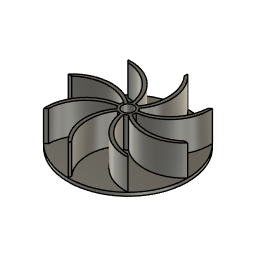
Rotor v3 (Autodesk Fusion 360 design; units mm, degrees)
Autodesk Fusion 360 part; units mm, degrees
sketch "Skizze1" plane through (0, 0, 0) normal (0, 0, 1) x (1, 0, 0)
  line L0 (-9.3696, -9.3689) -> (-13.6122, -5.1262) construction
  line L1 (-0.0006, -13.2498) -> (-4.5006, -13.2498) construction
  line L2 (-0.0004, 0) -> (18.7379, -18.7383)
  line L3 (-0.0004, 0) -> (18.7379, -18.7383) construction
  line L4 (-18.7387, -18.738) -> (-17.6781, -17.6774) construction
  arc A0 (-0.0006, -24.9998) -> (-0.0006, -1.4998) centre (13.0897, -13.2498) cw
  line L5 (13.2496, 0) -> (13.2496, -6) construction
  line L6 (-0.0006, -26.4998) -> (-0.0006, -24.9998) construction
  line L7 (-9.3696, 9.3692) -> (-5.1269, 13.6118) construction
  line L8 (-9.3696, 9.3692) -> (-5.1269, 13.6118) construction
  line L9 (-9.3696, 9.3692) -> (-6.1876, 12.5511) construction
  line L10 (-9.3696, 9.3692) -> (-6.1876, 12.5511) construction
  line L11 (-9.3696, 9.3692) -> (-6.1876, 12.5511) construction
  line L12 (-0.0004, 0) -> (18.7379, -18.7383) construction
  line L13 (-9.3696, 9.3692) -> (-5.1269, 13.6118) construction
  line L14 (9.3687, -9.3692) -> (5.1261, -13.6118) construction
  line L15 (9.3687, -9.3692) -> (6.1868, -12.5511) construction
  line L16 (9.3687, -9.3692) -> (6.1868, -12.5511) construction
  line L17 (9.3687, -9.3692) -> (5.1261, -13.6118) construction
  line L18 (9.3687, -9.3692) -> (6.1868, -12.5511) construction
  line L19 (-0.0006, -13.2498) -> (-6.0006, -13.2498) construction
  arc A1 (-17.6781, -17.6774) -> (-1.0611, -1.0604) centre (-0.1134, -18.6251) cw
  line L20 (9.3687, -9.3692) -> (6.1868, -12.5511) construction
  line L21 (9.3687, -9.3692) -> (5.1261, -13.6118) construction
  line L22 (9.3687, -9.3692) -> (5.1261, -13.6118) construction
  line L23 (9.3687, -9.3692) -> (5.1261, -13.6118) construction
  line L24 (9.3687, -9.3692) -> (6.1868, -12.5511) construction
  line L25 (-9.3696, -9.3689) -> (-12.5516, -6.1869) construction
  line L26 (-18.7387, 18.7383) -> (-17.6781, 17.6777) construction
  line L27 (-18.7387, 18.7383) -> (-17.6781, 17.6777) construction
  arc A2 (26.4996, 0) -> (-0.0004, 0) centre (13.2496, 11.6302) cw
  arc A3 (-25.0004, 0) -> (-1.5004, 0) centre (-13.2504, -13.0903) cw
  line L28 (-13.2504, 0) -> (-13.2504, 4.5) construction
  line L29 (-13.2504, 0) -> (-13.2504, 6) construction
  line L30 (-13.2504, 0) -> (-13.2504, 6) construction
  arc A4 (-25.0004, 0) -> (-1.5004, 0) centre (-13.2504, -13.0903) cw
  line L31 (-26.5004, 0) -> (-25.0004, 0) construction
  line L32 (-26.5004, 0) -> (-25.0004, 0) construction
  arc A5 (-17.6781, 17.6777) -> (-1.0611, 1.0607) centre (-18.6258, 0.1129) cw
  line L33 (-26.5004, 0) -> (-25.0004, 0) construction
  line L34 (-18.7387, 18.7383) -> (-17.6781, 17.6777) construction
  line L35 (-18.7387, 18.7383) -> (-17.6781, 17.6777) construction
  line L36 (-26.5004, 0) -> (-25.0004, 0) construction
  line L37 (-9.3696, 9.3692) -> (-5.1269, 13.6118) construction
  line L38 (-9.3696, 9.3692) -> (-6.1876, 12.5511) construction
  line L39 (-26.5004, 0) -> (-25.0004, 0) construction
  line L40 (-9.3696, 9.3692) -> (-5.1269, 13.6118) construction
  line L41 (-9.3696, 9.3692) -> (-6.1876, 12.5511) construction
  line L42 (-18.7387, 18.7383) -> (-17.6781, 17.6777) construction
  line L43 (-0.0004, 0) -> (-18.7387, 18.7383)
  line L44 (-0.0004, 0) -> (-1.0611, 1.0607) construction
  line L45 (-0.0004, 0) -> (-26.5004, 0)
  line L46 (-0.0004, 0) -> (-18.7387, 18.7383)
  line L47 (-0.0004, 0) -> (-1.0611, 1.0607) construction
  line L48 (-0.0004, 0) -> (-26.5004, 0)
  line L49 (-0.0004, 0) -> (13.2496, 0) construction
  line L50 (-0.0004, 0) -> (-26.5004, 0) construction
  line L51 (-0.0004, 0) -> (-9.3696, 9.3692) construction
  line L52 (-0.0004, 0) -> (-1.5004, 0) construction
  line L53 (-0.0004, 0) -> (-13.2504, 0) construction
  line L54 (-0.0004, 0) -> (26.4996, 0) construction
  arc A6 (-26.5004, 0) -> (-0.0004, 0) centre (-13.2504, -11.6302) cw
  line L55 (-0.0004, 0) -> (-26.5004, 0) construction
  line L56 (-0.0004, 0) -> (-9.3696, 9.3692) construction
  line L57 (-0.0004, 0) -> (-9.3696, 9.3692) construction
  line L58 (13.2496, 0) -> (13.2496, -4.5) construction
  line L59 (-0.0004, 0) -> (1.4996, 0) construction
  circle A7 centre (-0.0004, 0) radius 26.5
  line L60 (-0.0004, 0) -> (9.3687, -9.3692) construction
  line L61 (-0.0004, 0) -> (18.7379, -18.7383) construction
  line L62 (-0.0004, 0) -> (-9.3696, 9.3692) construction
  line L63 (-0.0002, -0.0002) -> (-0.0002, 26.4998)
  line L64 (-0.0004, 0) -> (-1.0611, 1.0607) construction
  circle A8 centre (-0.0004, 0) radius 2.55
  arc A9 (-18.7387, 18.7383) -> (-0.0004, 0) centre (-17.5934, 1.1454) cw
  line L65 (-0.0004, 0) -> (1.4996, 0) construction
  line L66 (-0.0004, 0) -> (26.4996, 0)
  line L67 (-0.0004, 0) -> (13.2496, 0) construction
  line L68 (-0.0004, 0) -> (26.4996, 0)
  line L69 (-0.0004, 0) -> (-1.0611, 1.0607) construction
  arc A10 (-0.0002, 24.9998) -> (-0.0002, 1.4998) centre (-13.0905, 13.2498) cw
  line L70 (-0.0004, 0.0003) -> (-9.3696, -9.3689) construction
  line L71 (-0.0004, 0) -> (-18.7387, 18.7383) construction
  line L72 (-0.0004, -0.0003) -> (9.3687, 9.3689) construction
  arc A11 (-0.0002, 26.4998) -> (-0.0002, -0.0002) centre (-11.6304, 13.2498) cw
  line L73 (-0.0004, 0) -> (-26.5004, 0)
  line L74 (-0.0004, 0) -> (-26.5004, 0)
  line L75 (-0.0004, 0) -> (-26.5004, 0) construction
  arc A12 (-26.5004, 0) -> (-0.0004, 0) centre (-13.2504, -11.6302) cw
  arc A13 (-18.7387, 18.7383) -> (-0.0004, 0) centre (-17.5934, 1.1454) cw
  line L76 (-0.0004, 0) -> (26.4996, 0) construction
  line L77 (-0.0004, 0) -> (26.4996, 0) construction
  line L78 (-0.0004, 0) -> (-26.5004, 0) construction
  line L79 (-0.0004, 0) -> (-26.5004, 0)
  arc A14 (18.7379, 18.738) -> (-0.0004, -0.0003) centre (1.1449, 17.5927) cw
  line L80 (-0.0004, 0) -> (1.4996, 0) construction
  arc A15 (-26.5004, 0) -> (-0.0004, 0) centre (-13.2504, -11.6302) cw
  line L81 (-0.0004, 0) -> (-18.7387, 18.7383) construction
  line L82 (-0.0004, 0) -> (26.4996, 0)
  line L83 (-0.0004, 0) -> (-26.5004, 0) construction
  line L84 (-0.0004, 0) -> (26.4996, 0)
  arc A16 (-18.7387, 18.7383) -> (-0.0004, 0) centre (-17.5934, 1.1454) cw
  arc A17 (-18.7387, 18.7383) -> (-0.0004, 0) centre (-17.5934, 1.1454) cw
  line L85 (-0.0004, 0) -> (-1.5004, 0) construction
  line L86 (-0.0004, 0) -> (-13.2504, 0) construction
  line L87 (-0.0004, 0) -> (-1.5004, 0) construction
  line L88 (-0.0004, 0) -> (26.4996, 0) construction
  line L89 (-0.0004, 0) -> (-13.2504, 0) construction
  line L90 (-0.0004, 0) -> (1.4996, 0) construction
  arc A18 (-18.7387, 18.7383) -> (-0.0004, 0) centre (-17.5934, 1.1454) cw
  line L91 (-0.0004, 0) -> (13.2496, 0) construction
  line L92 (-0.0004, 0) -> (-18.7387, 18.7383)
  line L93 (-0.0004, 0) -> (-18.7387, 18.7383) construction
  line L94 (-0.0004, 0) -> (26.4996, 0) construction
  line L95 (-0.0004, 0) -> (-1.5004, 0) construction
  line L96 (-0.0004, 0) -> (-1.5004, 0) construction
  line L97 (-0.0004, 0) -> (-18.7387, 18.7383) construction
  arc A19 (-26.5004, 0) -> (-0.0004, 0) centre (-13.2504, -11.6302) cw
  line L98 (-0.0004, 0) -> (1.4996, 0) construction
  line L99 (-0.0004, 0) -> (-13.2504, 0) construction
  arc A20 (-26.5004, 0) -> (-0.0004, 0) centre (-13.2504, -11.6302) cw
  line L100 (-0.0004, 0) -> (-18.7387, 18.7383)
  line L101 (-0.0004, 0) -> (-18.7387, 18.7383) construction
  line L102 (-0.0004, 0) -> (-9.3696, 9.3692) construction
  line L103 (-0.0004, 0) -> (-13.2504, 0) construction
  line L104 (-0.0004, 0) -> (-18.7387, 18.7383)
  line L105 (-0.0004, 0) -> (-1.0611, 1.0607) construction
  line L106 (-0.0004, 0) -> (13.2496, 0) construction
  line L107 (-0.0004, 0) -> (13.2496, 0) construction
  line L108 (-0.0004, 0) -> (26.4996, 0)
  arc A21 (17.6773, -17.6777) -> (1.0602, -1.0607) centre (18.625, -0.1129) cw
  line L109 (18.7379, -18.7383) -> (17.6773, -17.6777) construction
  arc A22 (17.6773, -17.6777) -> (1.0602, -1.0607) centre (18.625, -0.1129) cw
  arc A23 (17.6773, -17.6777) -> (1.0602, -1.0607) centre (18.625, -0.1129) cw
  arc A24 (17.6773, -17.6777) -> (1.0602, -1.0607) centre (18.625, -0.1129) cw
  arc A25 (17.6773, -17.6777) -> (1.0602, -1.0607) centre (18.625, -0.1129) cw
  line L110 (18.7379, -18.7383) -> (17.6773, -17.6777) construction
  line L111 (18.7379, -18.7383) -> (17.6773, -17.6777) construction
  line L112 (18.7379, -18.7383) -> (17.6773, -17.6777) construction
  line L113 (18.7379, -18.7383) -> (17.6773, -17.6777) construction
  arc A26 (-25.0004, 0) -> (-1.5004, 0) centre (-13.2504, -13.0903) cw
  arc A27 (-17.6781, 17.6777) -> (-1.0611, 1.0607) centre (-18.6258, 0.1129) cw
  line L114 (13.2496, 0) -> (13.2496, -4.5) construction
  line L115 (13.2496, 0) -> (13.2496, -6) construction
  arc A28 (26.4996, 0) -> (-0.0004, 0) centre (13.2496, 11.6302) cw
  line L116 (-13.2504, 0) -> (-13.2504, 4.5) construction
  line L117 (-0.0004, 0) -> (18.7379, -18.7383) construction
  arc A29 (-17.6781, 17.6777) -> (-1.0611, 1.0607) centre (-18.6258, 0.1129) cw
  arc A30 (-18.7387, -18.738) -> (-0.0004, 0.0003) centre (-1.1458, -17.5927) cw
  line L118 (-13.2504, 0) -> (-13.2504, 4.5) construction
  arc A31 (-25.0004, 0) -> (-1.5004, 0) centre (-13.2504, -13.0903) cw
  line L119 (-13.2504, 0) -> (-13.2504, 6) construction
  line L120 (-0.0004, 0) -> (9.3687, -9.3692) construction
  arc A32 (-17.6781, 17.6777) -> (-1.0611, 1.0607) centre (-18.6258, 0.1129) cw
  line L121 (-13.2504, 0) -> (-13.2504, 6) construction
  arc A33 (-17.6781, 17.6777) -> (-1.0611, 1.0607) centre (-18.6258, 0.1129) cw
  arc A34 (26.4996, 0) -> (-0.0004, 0) centre (13.2496, 11.6302) cw
  arc A35 (18.7379, -18.7383) -> (-0.0004, 0) centre (17.5925, -1.1454) cw
  circle A36 centre (-0.0004, 0) radius 3.5
  line L122 (-13.2504, 0) -> (-13.2504, 6) construction
  line L123 (-0.0004, 0.0003) -> (-18.7387, -18.738)
  line L124 (13.2496, 0) -> (13.2496, -4.5) construction
  line L125 (-0.0004, 0) -> (18.7379, -18.7383) construction
  line L126 (-13.2504, 0) -> (-13.2504, 4.5) construction
  arc A37 (-25.0004, 0) -> (-1.5004, 0) centre (-13.2504, -13.0903) cw
  line L127 (-13.2504, 0) -> (-13.2504, 4.5) construction
  line L128 (-0.0004, 0) -> (18.7379, -18.7383)
  line L129 (-0.0004, 0) -> (18.7379, -18.7383)
  line L130 (-0.0004, 0) -> (1.0602, -1.0607) construction
  line L131 (-0.0004, -0.0003) -> (1.0602, 1.0604) construction
  arc A38 (24.9996, 0) -> (1.4996, 0) centre (13.2496, 13.0903) cw
  line L132 (26.4996, 0) -> (24.9996, 0) construction
  line L133 (13.2496, 0) -> (13.2496, -4.5) construction
  arc A39 (-0.0006, -26.4998) -> (-0.0006, 0.0002) centre (11.6296, -13.2498) cw
  line L134 (-0.0002, 26.4998) -> (-0.0002, 24.9998) construction
  arc A40 (18.7379, -18.7383) -> (-0.0004, 0) centre (17.5925, -1.1454) cw
  line L135 (13.2496, 0) -> (13.2496, -4.5) construction
  line L136 (26.4996, 0) -> (24.9996, 0) construction
  line L137 (-0.0006, 0.0002) -> (-0.0006, -1.4998) construction
  arc A41 (26.4996, 0) -> (-0.0004, 0) centre (13.2496, 11.6302) cw
  line L138 (-0.0006, 0.0002) -> (-0.0006, -26.4998) construction
  line L139 (13.2496, 0) -> (13.2496, -6) construction
  line L140 (26.4996, 0) -> (24.9996, 0) construction
  line L141 (-0.0004, 0) -> (1.0602, -1.0607) construction
  line L142 (-0.0002, -0.0002) -> (-0.0002, 1.4998) construction
  line L143 (-0.0004, 0) -> (18.7379, -18.7383)
  line L144 (-0.0004, 0) -> (9.3687, -9.3692) construction
  arc A42 (24.9996, 0) -> (1.4996, 0) centre (13.2496, 13.0903) cw
  line L145 (-0.0004, 0) -> (1.0602, -1.0607) construction
  line L146 (-0.0006, 0.0002) -> (-0.0006, -26.4998)
  line L147 (26.4996, 0) -> (24.9996, 0) construction
  line L148 (-0.0004, 0) -> (1.0602, -1.0607) construction
  line L149 (26.4996, 0) -> (24.9996, 0) construction
  arc A43 (18.7379, -18.7383) -> (-0.0004, 0) centre (17.5925, -1.1454) cw
  line L150 (-0.0002, -0.0002) -> (-0.0002, 13.2498) construction
  arc A44 (17.6773, 17.6774) -> (1.0602, 1.0604) centre (0.1125, 18.6251) cw
  arc A45 (18.7379, -18.7383) -> (-0.0004, 0) centre (17.5925, -1.1454) cw
  arc A46 (26.4996, 0) -> (-0.0004, 0) centre (13.2496, 11.6302) cw
  line L151 (18.7379, 18.738) -> (17.6773, 17.6774) construction
  line L152 (-0.0004, 0) -> (1.0602, -1.0607) construction
  line L153 (-0.0004, 0.0003) -> (-1.0611, -1.0604) construction
  line L154 (-0.0004, 0.0003) -> (-18.7387, -18.738) construction
  line L155 (-0.0004, 0) -> (9.3687, -9.3692) construction
  line L156 (-0.0004, 0) -> (9.3687, -9.3692) construction
  line L157 (-0.0002, 13.2498) -> (4.4998, 13.2498) construction
  line L158 (-0.0006, 0.0002) -> (-0.0006, -13.2498) construction
  line L159 (-0.0002, -0.0002) -> (-0.0002, 26.4998) construction
  arc A47 (24.9996, 0) -> (1.4996, 0) centre (13.2496, 13.0903) cw
  line L160 (9.3687, 9.3689) -> (13.6114, 5.1262) construction
  arc A48 (18.7379, -18.7383) -> (-0.0004, 0) centre (17.5925, -1.1454) cw
  arc A49 (24.9996, 0) -> (1.4996, 0) centre (13.2496, 13.0903) cw
  line L161 (9.3687, 9.3689) -> (12.5507, 6.1869) construction
  line L162 (13.2496, 0) -> (13.2496, -6) construction
  line L163 (-0.0002, 13.2498) -> (5.9998, 13.2498) construction
  line L164 (-0.0004, -0.0003) -> (18.7379, 18.738) construction
  line L165 (-0.0004, -0.0003) -> (18.7379, 18.738)
  line L166 (-0.0004, 0) -> (18.7379, -18.7383)
  line L167 (13.2496, 0) -> (13.2496, -6) construction
  arc A50 (24.9996, 0) -> (1.4996, 0) centre (13.2496, 13.0903) cw
  point P0 (-0.0006, 0.0002)
  point P1 (-0.0004, 0)
  point P2 (-0.0004, 0)
  point P3 (-0.0006, 0.0002)
  point P4 (-0.0006, 0.0002)
  point P5 (-0.0004, 0)
  point P6 (-0.0004, 0)
  point P7 (-0.0004, 0)
  point P8 (-0.0004, 0)
  point P9 (-0.0004, 0)
  point P10 (-0.0004, 0)
  point P11 (-0.0004, 0)
  point P12 (-0.0002, -0.0002)
  point P13 (-0.0002, -0.0002)
  point P14 (-0.0004, 0)
  point P15 (-0.0004, 0)
  point P16 (-0.0004, 0)
  point P17 (-0.0002, -0.0002)
  point P18 (-0.0002, -0.0002)
  point P19 (-0.0002, -0.0002)
  point P20 (-0.0004, -0.0003)
  point P21 (-0.0004, 0)
  point P22 (-0.0004, -0.0003)
  point P23 (-0.0004, -0.0003)
  point P24 (-0.0004, 0)
  point P25 (-0.0004, 0)
  point P26 (-0.0004, 0)
  point P27 (-0.0004, 0)
  point P28 (-0.0004, -0.0003)
  point P29 (-0.0004, 0)
  point P30 (-0.0004, 0)
  point P31 (-0.0004, 0)
  point P32 (-0.0004, 0)
  point P33 (-0.0004, 0)
  point P34 (-0.0004, 0)
  point P35 (-0.0004, 0)
  point P36 (-0.0004, 0)
  point P37 (-0.0004, 0)
  point P38 (-0.0004, 0)
  point P39 (-0.0004, 0)
  point P40 (-0.0004, 0)
  point P41 (-0.0004, 0)
  point P42 (-0.0004, 0)
  point P43 (-0.0004, 0)
  point P44 (-0.0004, 0)
  point P45 (-0.0004, 0)
  point P46 (-0.0004, 0)
  point P47 (-0.0004, 0)
  point P48 (-0.0004, 0)
  point P49 (-0.0004, 0)
  point P50 (-0.0004, 0)
  point P51 (-0.0004, 0)
  point P52 (-0.0004, 0)
  point P53 (-0.0004, 0)
  point P54 (-0.0004, 0)
  point P55 (-0.0004, 0)
  point P56 (-0.0004, 0.0003)
  point P57 (-0.0004, 0.0003)
  point P58 (-0.0004, 0)
  point P59 (-0.0004, 0)
  point P60 (-0.0004, 0.0003)
  point P61 (-0.0004, 0.0003)
  point P62 (-0.0004, 0)
  point P63 (-0.0004, 0)
  point P64 (-0.0004, 0)
  point P65 (-0.0004, 0.0003)
  point P66 (-0.0004, 0)
  point P67 (-0.0004, 0)
  point P68 (-0.0004, 0)
  point P69 (-0.0004, 0)
  point P70 (-0.0004, 0)
  point P71 (-0.0004, 0)
  point P72 (-0.0004, 0)
  point P73 (-0.0004, 0)
  point P74 (-0.0004, 0)
  point P75 (-0.0004, 0)
  point P76 (-0.0004, 0)
  point P77 (-0.0004, 0)
  point P78 (-0.0004, -0.0003)
  point P79 (-0.0004, 0)
  point P80 (-0.0004, 0)
  point P81 (-0.0004, 0)
  point P82 (-0.0004, 0)
  point P83 (-0.0004, 0)
  point P84 (-0.0004, 0)
  point P85 (-0.0004, 0)
  point P86 (-0.0004, 0)
  point P87 (-0.0004, 0)
  point P88 (-0.0006, 0.0002)
  point P89 (-0.0004, 0)
  point P90 (-0.0004, 0)
  point P91 (-0.0004, 0)
  point P92 (-0.0006, 0.0002)
  point P93 (-0.0004, 0)
  point P94 (-0.0004, 0)
  dimension "d135" = 53
  dimension "d136" = 13.25
  dimension "d137" = 6
  dimension "d138" = 4.5
  dimension "d139" = 1.5
  dimension "d140" = 1.5
  dimension "d141" = 13.25
  dimension "d142" = 6
  dimension "d143" = 4.5
  dimension "d144" = 1.5
  dimension "d145" = 1.5
  dimension "d146" = 13.25
  dimension "d147" = 6
  dimension "d148" = 4.5
  dimension "d149" = 1.5
  dimension "d150" = 1.5
  dimension "d151" = 13.25
  dimension "d152" = 6
  dimension "d153" = 4.5
  dimension "d154" = 1.5
  dimension "d155" = 1.5
  dimension "d156" = 13.25
  dimension "d157" = 6
  dimension "d158" = 4.5
  dimension "d159" = 1.5
  dimension "d160" = 1.5
  dimension "d161" = 13.25
  dimension "d162" = 6
  dimension "d163" = 4.5
  dimension "d164" = 1.5
  dimension "d165" = 1.5
  dimension "d166" = 13.25
  dimension "d167" = 6
  dimension "d168" = 4.5
  dimension "d169" = 1.5
  dimension "d170" = 1.5
  dimension "d171" = 13.25
  dimension "d172" = 6
  dimension "d173" = 4.5
  dimension "d174" = 1.5
  dimension "d175" = 1.5
  dimension "d176" = 13.25
  dimension "d177" = 6
  dimension "d178" = 4.5
  dimension "d179" = 1.5
  dimension "d180" = 1.5
  dimension "d181" = 13.25
  dimension "d182" = 6
  dimension "d183" = 4.5
  dimension "d184" = 1.5
  dimension "d185" = 1.5
  dimension "d186" = 13.25
  dimension "d187" = 6
  dimension "d188" = 4.5
  dimension "d189" = 1.5
  dimension "d190" = 1.5
  dimension "d191" = 13.25
  dimension "d192" = 6
  dimension "d193" = 4.5
  dimension "d194" = 1.5
  dimension "d195" = 1.5
  dimension "d196" = 13.25
  dimension "d197" = 6
  dimension "d198" = 4.5
  dimension "d199" = 1.5
  dimension "d200" = 1.5
  dimension "d201" = 13.25
  dimension "d202" = 6
  dimension "d203" = 4.5
  dimension "d204" = 1.5
  dimension "d205" = 1.5
  dimension "d206" = 13.25
  dimension "d207" = 6
  dimension "d208" = 4.5
  dimension "d209" = 1.5
  dimension "d210" = 1.5
  dimension "d211" = 13.25
  dimension "d212" = 6
  dimension "d213" = 4.5
  dimension "d214" = 1.5
  dimension "d215" = 1.5
  dimension "d216" = 13.25
  dimension "d217" = 6
  dimension "d218" = 4.5
  dimension "d219" = 1.5
  dimension "d220" = 1.5
  dimension "d221" = 13.25
  dimension "d222" = 6
  dimension "d223" = 4.5
  dimension "d224" = 1.5
  dimension "d225" = 1.5
  dimension "d226" = 13.25
  dimension "d227" = 6
  dimension "d228" = 4.5
  dimension "d229" = 1.5
  dimension "d230" = 1.5
  dimension "d231" = 13.25
  dimension "d232" = 6
  dimension "d233" = 4.5
  dimension "d234" = 1.5
  dimension "d235" = 1.5
  dimension "d236" = 13.25
  dimension "d237" = 6
  dimension "d238" = 4.5
  dimension "d239" = 1.5
  dimension "d240" = 1.5
  dimension "d241" = 13.25
  dimension "d242" = 6
  dimension "d243" = 4.5
  dimension "d244" = 1.5
  dimension "d245" = 1.5
  dimension "d246" = 13.25
  dimension "d247" = 6
  dimension "d248" = 4.5
  dimension "d249" = 1.5
  dimension "d250" = 1.5
  dimension "d251" = 13.25
  dimension "d252" = 6
  dimension "d253" = 4.5
  dimension "d254" = 1.5
  dimension "d255" = 1.5
  dimension "d256" = 5.1
  dimension "d257" = 7
  constraint coincident P94 P93
  constraint parallel L48 L78
  constraint midpoint L28.start L78
  constraint perpendicular L48 L121
  constraint coincident L29.end A12
  constraint perpendicular L89 L126
  constraint perpendicular L85 L126
  constraint coincident A3.start L78
  constraint coincident L28.end A4
  constraint parallel L50 L79
  constraint midpoint L28.start L50
  constraint perpendicular L79 L119
  constraint coincident L29.end A6
  constraint perpendicular L103 L118
  constraint perpendicular L96 L118
  constraint coincident A3.start L50
  constraint coincident L28.end A3
  constraint coincident P19 P18
  constraint parallel L63 L159
  constraint midpoint L150.end L159
  constraint perpendicular L63 L163
  constraint coincident L163.end A11
  constraint perpendicular L150 L157
  constraint perpendicular L142 L157
  constraint coincident A10.start L159
  constraint coincident L157.end A10
  constraint parallel L73 L75
  constraint midpoint L28.start L75
  constraint perpendicular L30 L73
  constraint coincident L29.end A20
  constraint perpendicular L86 L116
  constraint perpendicular L95 L116
  constraint coincident A3.start L75
  constraint coincident L28.end A26
  constraint parallel L74 L83
  constraint midpoint L28.start L83
  constraint perpendicular L74 L122
  constraint coincident L29.end A15
  constraint perpendicular L99 L127
  constraint perpendicular L52 L127
  constraint coincident A3.start L83
  constraint coincident L28.end A37
  constraint parallel L45 L55
  constraint midpoint L28.start L55
  constraint perpendicular L29 L45
  constraint coincident L29.end A19
  constraint perpendicular L28 L53
  constraint perpendicular L28 L87
  constraint coincident A3.start L55
  constraint coincident L28.end A31
  constraint parallel L68 L76
  constraint midpoint L5.start L76
  constraint perpendicular L68 L139
  constraint coincident L5.end A41
  constraint perpendicular L106 L124
  constraint perpendicular L90 L124
  constraint coincident A38.start L76
  constraint coincident L58.end A42
  constraint parallel L82 L88
  constraint midpoint L5.start L88
  constraint perpendicular L82 L167
  constraint coincident L5.end A2
  constraint perpendicular L91 L135
  constraint perpendicular L59 L135
  constraint coincident A38.start L88
  constraint coincident L58.end A49
  constraint coincident P92 P88
  constraint parallel L138 L146
  constraint midpoint L1.start L138
  constraint perpendicular L19 L146
  constraint coincident L19.end A39
  constraint perpendicular L1 L158
  constraint perpendicular L1 L137
  constraint coincident A0.start L138
  constraint coincident L1.end A0
  constraint parallel L54 L66
  constraint midpoint L5.start L54
  constraint perpendicular L66 L115
  constraint coincident L5.end A34
  constraint perpendicular L67 L114
  constraint perpendicular L80 L114
  constraint coincident A38.start L54
  constraint coincident L58.end A38
  constraint parallel L84 L94
  constraint midpoint L5.start L94
  constraint perpendicular L84 L162
  constraint coincident L5.end A28
  constraint perpendicular L49 L58
  constraint perpendicular L58 L98
  constraint coincident A38.start L94
  constraint coincident L58.end A47
  constraint parallel L77 L108
  constraint midpoint L5.start L77
  constraint perpendicular L5 L108
  constraint coincident L5.end A46
  constraint perpendicular L107 L133
  constraint perpendicular L65 L133
  constraint coincident A38.start L77
  constraint coincident L58.end A50
  constraint parallel L71 L104
  constraint midpoint L7.start L71
  constraint perpendicular L37 L104
  constraint coincident L7.end A9
  constraint perpendicular L41 L102
  constraint perpendicular L41 L44
  constraint coincident L26.end L71
  constraint coincident L9.end A27
  constraint parallel L46 L93
  constraint midpoint L7.start L93
  constraint perpendicular L7 L46
  constraint coincident L7.end A18
  constraint perpendicular L38 L51
  constraint perpendicular L38 L105
  constraint coincident L26.end L93
  constraint coincident L9.end A32
  constraint coincident P78 P28
  constraint parallel L164 L165
  constraint midpoint L72.end L164
  constraint perpendicular L160 L165
  constraint coincident L160.end A14
  constraint perpendicular L72 L161
  constraint perpendicular L131 L161
  constraint coincident A44.start L164
  constraint coincident L161.end A44
  constraint parallel L81 L92
  constraint midpoint L7.start L81
  constraint perpendicular L40 L92
  constraint coincident L7.end A17
  constraint perpendicular L9 L56
  constraint perpendicular L9 L69
  constraint coincident L26.end L81
  constraint coincident L9.end A5
  constraint parallel L43 L101
  constraint midpoint L7.start L101
  constraint perpendicular L8 L43
  constraint coincident L7.end A13
  constraint perpendicular L11 L62
  constraint perpendicular L11 L47
  constraint coincident L26.end L101
  constraint coincident L9.end A33
  constraint parallel L97 L100
  constraint midpoint L7.start L97
  constraint perpendicular L13 L100
  constraint coincident L7.end A16
  constraint perpendicular L10 L57
  constraint perpendicular L10 L64
  constraint coincident L26.end L97
  constraint coincident L9.end A29
  constraint parallel L12 L129
  constraint midpoint L14.start L12
  constraint perpendicular L23 L129
  constraint coincident L14.end A43
  constraint perpendicular L16 L144
  constraint perpendicular L16 L148
  constraint coincident A21.start L12
  constraint coincident L15.end A21
  constraint parallel L2 L125
  constraint midpoint L14.start L125
  constraint perpendicular L2 L22
  constraint coincident L14.end A48
  constraint perpendicular L18 L156
  constraint perpendicular L18 L141
  constraint coincident A21.start L125
  constraint coincident L15.end A22
  constraint coincident P65 P61
  constraint parallel L123 L154
  constraint midpoint L0.start L154
  constraint perpendicular L0 L123
  constraint coincident L0.end A30
  constraint perpendicular L25 L70
  constraint perpendicular L25 L153
  constraint coincident L4.end L154
  constraint coincident L25.end A1
  constraint parallel L117 L166
  constraint midpoint L14.start L117
  constraint perpendicular L21 L166
  constraint coincident L14.end A45
  constraint perpendicular L20 L155
  constraint perpendicular L20 L130
  constraint coincident A21.start L117
  constraint coincident L15.end A23
  constraint parallel L3 L143
  constraint midpoint L14.start L3
  constraint perpendicular L14 L143
  constraint coincident L14.end A40
  constraint perpendicular L24 L60
  constraint perpendicular L24 L145
  constraint coincident A21.start L3
  constraint coincident L15.end A25
  constraint parallel L61 L128
  constraint midpoint L14.start L61
  constraint perpendicular L17 L128
  constraint coincident L14.end A35
  constraint perpendicular L15 L120
  constraint perpendicular L15 L152
  constraint coincident A21.start L61
  constraint coincident L15.end A24
  measures "d135" diameter of A7
  measures "d136" distance of P94 L28.start
  measures "d137" distance of L29.end L28.start
  measures "d138" distance of L28.end L28.start
  measures "d139" distance of A3.end P94
  measures "d140" distance of L31.start A3.start
  measures "d141" distance of L28.start P94
  measures "d142" distance of L29.end L28.start
  measures "d143" distance of L28.start L28.end
  measures "d144" distance of P94 A3.end
  measures "d145" distance of L31.start A3.start
  measures "d146" distance of P19 L150.end
  measures "d147" distance of L163.end L150.end
  measures "d148" distance of L157.end L150.end
  measures "d149" distance of A10.end P19
  measures "d150" distance of A10.start L63.end
  measures "d151" distance of P94 L28.start
  measures "d152" distance of L29.end L28.start
  measures "d153" distance of L28.start L28.end
  measures "d154" distance of P94 A3.end
  measures "d155" distance of A3.start L31.start
  measures "d156" distance of L28.start P94
  measures "d157" distance of L28.start L29.end
  measures "d158" distance of L28.end L28.start
  measures "d159" distance of P94 A3.end
  measures "d160" distance of A3.start L31.start
  measures "d161" distance of P94 L28.start
  measures "d162" distance of L29.end L28.start
  measures "d163" distance of L28.end L28.start
  measures "d164" distance of P94 A3.end
  measures "d165" distance of L31.start A3.start
  measures "d166" distance of P94 L5.start
  measures "d167" distance of L5.end L5.start
  measures "d168" distance of L58.end L5.start
  measures "d169" distance of L59.end P94
  measures "d170" distance of A38.start A2.start
  measures "d171" distance of P94 L5.start
  measures "d172" distance of L5.end L5.start
  measures "d173" distance of L58.end L5.start
  measures "d174" distance of P94 L59.end
  measures "d175" distance of A2.start A38.start
  measures "d176" distance of P92 L1.start
  measures "d177" distance of L19.end L1.start
  measures "d178" distance of L1.start L1.end
  measures "d179" distance of A0.end P92
  measures "d180" distance of L6.start A0.start
  measures "d181" distance of P94 L5.start
  measures "d182" distance of L5.end L5.start
  measures "d183" distance of L58.end L5.start
  measures "d184" distance of P94 L59.end
  measures "d185" distance of A38.start A2.start
  measures "d186" distance of P94 L5.start
  measures "d187" distance of L5.start L5.end
  measures "d188" distance of L58.end L5.start
  measures "d189" distance of P94 L59.end
  measures "d190" distance of A2.start A38.start
  measures "d191" distance of L5.start P94
  measures "d192" distance of L5.end L5.start
  measures "d193" distance of L5.start L58.end
  measures "d194" distance of P94 L59.end
  measures "d195" distance of A38.start A2.start
  measures "d196" distance of P94 L7.start
  measures "d197" distance of L7.end L7.start
  measures "d198" distance of L9.end L7.start
  measures "d199" distance of A5.end P94
  measures "d200" distance of L26.start L26.end
  measures "d201" distance of P94 L7.start
  measures "d202" distance of L7.end L7.start
  measures "d203" distance of L7.start L9.end
  measures "d204" distance of P94 A5.end
  measures "d205" distance of L26.start L26.end
  measures "d206" distance of P78 L72.end
  measures "d207" distance of L160.end L72.end
  measures "d208" distance of L161.end L72.end
  measures "d209" distance of L131.end P28
  measures "d210" distance of A14.start A44.start
  measures "d211" distance of P94 L7.start
  measures "d212" distance of L7.start L7.end
  measures "d213" distance of L9.end L7.start
  measures "d214" distance of A5.end P94
  measures "d215" distance of L26.end L26.start
  measures "d216" distance of L7.start P94
  measures "d217" distance of L7.start L7.end
  measures "d218" distance of L7.start L9.end
  measures "d219" distance of P94 A5.end
  measures "d220" distance of L26.end L26.start
  measures "d221" distance of P94 L7.start
  measures "d222" distance of L7.end L7.start
  measures "d223" distance of L9.end L7.start
  measures "d224" distance of P94 A5.end
  measures "d225" distance of L26.end L26.start
  measures "d226" distance of P94 L14.start
  measures "d227" distance of L14.end L14.start
  measures "d228" distance of L14.start L15.end
  measures "d229" distance of P94 A21.end
  measures "d230" distance of A21.start L2.end
  measures "d231" distance of L14.start P94
  measures "d232" distance of L14.start L14.end
  measures "d233" distance of L14.start L15.end
  measures "d234" distance of P94 A21.end
  measures "d235" distance of L2.end A21.start
  measures "d236" distance of P65 L0.start
  measures "d237" distance of L0.start L0.end
  measures "d238" distance of L0.start L25.end
  measures "d239" distance of P65 A1.end
  measures "d240" distance of L4.end L4.start
  measures "d241" distance of L14.start P94
  measures "d242" distance of L14.end L14.start
  measures "d243" distance of L15.end L14.start
  measures "d244" distance of A21.end P94
  measures "d245" distance of L2.end A21.start
  measures "d246" distance of L14.start P94
  measures "d247" distance of L14.start L14.end
  measures "d248" distance of L14.start L15.end
  measures "d249" distance of P94 A21.end
  measures "d250" distance of L2.end A21.start
  measures "d251" distance of L14.start P94
  measures "d252" distance of L14.start L14.end
  measures "d253" distance of L14.start L15.end
  measures "d254" distance of A21.end P94
  measures "d255" distance of A21.start L2.end
  measures "d256" diameter of A8
  measures "d257" diameter of A36
extrude "Extrusion1" add sketch "Skizze1" along normal blind 1.5 contours L2 A21 A22 A23 A24 A25 A36 L128 L129 L143 L166 | A5 L43 L46 L92 L100 L104 A27 A29 A32 A33 A36 | L63 A10 A36 | A36 A44 L165 | L66 L68 L82 L84 L108 A36 A38 A42 A47 A49 A50 | A3 A4 L45 L48 L73 L74 L79 A26 A31 A36 A37 | A0 A36 L146 | A1 A36 L123 | L2 A2 A7 A28 A34 A36 L128 L129 A41 L143 A46 L166 | A7 A35 A36 A40 L146 A43 A45 A48 | L43 L46 A6 A7 A12 A15 L92 A19 A20 L100 L104 A36 | L45 L48 A7 L73 L74 L79 A30 A36 | A7 L63 A9 A13 A16 A17 A18 A36 | A7 A11 A36 L165 | A7 L66 L68 A14 L82 L84 L108 A36 | A7 A36 L123 A39
extrude "Extrusion3" add sketch "Skizze1" along normal blind 15 contours A8 A21 A22 A23 A24 A25 A35 A36 A40 A43 A45 A48 | L2 A8 A21 A22 A23 A24 A25 A36 L128 L129 L143 L166 | A5 L43 L46 A8 L92 L100 L104 A27 A29 A32 A33 A36 | A5 A8 A9 A13 A16 A17 A18 A27 A29 A32 A33 A36 | A8 A10 A11 A36 | L63 A8 A10 A36 | A8 A14 A36 A44 | A8 A36 A44 L165 | A2 A8 A28 A34 A36 A38 A41 A42 A46 A47 A49 A50 | A8 L66 L68 L82 L84 L108 A36 A38 A42 A47 A49 A50 | A3 A4 L45 L48 A8 L73 L74 L79 A26 A31 A36 A37 | A3 A4 A6 A8 A12 A15 A19 A20 A26 A31 A36 A37 | A0 A8 A36 L146 | A0 A8 A36 A39 | A1 A8 A36 L123 | A1 A8 A30 A36 | L2 A2 A8 A28 A34 A36 L128 L129 A41 L143 A46 L166 | A8 A35 A36 A40 L146 A43 A45 A48 | L2 A21 A22 A23 A24 A25 A35 A36 L128 L129 A40 L143 A43 A45 A48 L166 | L43 L46 A6 A8 A12 A15 L92 A19 A20 L100 L104 A36 | L45 L48 A8 L73 L74 L79 A30 A36 | A5 L43 L46 A9 A13 A16 A17 A18 L92 L100 L104 A27 A29 A32 A33 A36 | L63 A8 A9 A13 A16 A17 A18 A36 | A8 A11 A36 L165 | L63 A10 A11 A36 | A8 L66 L68 A14 L82 L84 L108 A36 | A14 A36 A44 L165 | A2 L66 L68 L82 L84 L108 A28 A34 A36 A38 A41 A42 A46 A47 A49 A50 | A3 A4 L45 L48 A6 L73 L74 A12 L79 A15 A19 A20 A26 A31 A36 A37 | A0 A36 A39 L146 | A8 A36 L123 A39 | A1 A30 A36 L123
